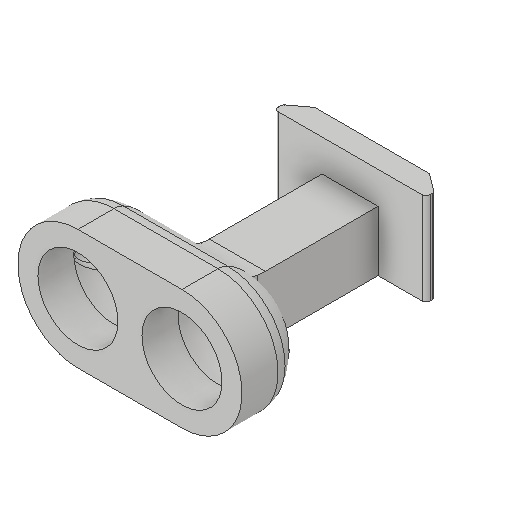
# Autodesk Inventor part: Engate CNMF NEM355-5.50
Saved by Autodesk Inventor 2026.2 (Build 302298010, 298A)
## iProperties
Manager: MANUTENÇÃO GUIFÕES - CP
Company: CP
Created: 2025-09-02
Part Number: Engate CNMF NEM355-5.50
Project: 0.00 0000/00
Checked By: PMFIGUEIREDO
Engr Approved By: JSSILVA
Material: Generic
Description: NOME DA PEÇA
Document SubType Name: Modeling
Designer: TPMIRANDA
Engineer: ISO 2768 - m K
Authority: Nº DESENHO PELO QUAL FOI SUBSITUIDO
Stock Number: 00000-000
Density: 1 g/cm^3
Appearance: Default
Distância: 5,500 mm
Title: UME 3400
Subject: CAIXA, INTERIOR, SUPORTE,
Author: TPMIRANDA
Keywords: Caixa de comentários. Substituir texto, ou eliminar.
Comments: UQE2300 UQE2400 UTE2240 UDD9630 CARRUAGENS SIMAFE CARRUAGENS CAF CARRUAGENS ARCO
Revision Number: Nº DESENHO QUE SUBSTITUI
Autodesk Inventor part; units mm, degrees
ref_plane "XY Plane" through (0, 0, 0) normal (0, 0, 1) x (1, 0, 0)
sketch "Sketch1" plane through (0, 0, 0) normal (0, 0, 1) x (1, 0, 0)
  line L0 (-1.3, 0) -> (1.3, 0) construction
  line L1 (1.3, 0) -> (1.3, 2)
  line L2 (1.3, 0) -> (2.8, 0)
  line L3 (2.8, 0) -> (2.8, 0.9)
  line L4 (2.3, 0) -> (2.3, 0.9)
  arc A0 (2.8, 0.9) -> (2.7412, 1.1353) centre (2.3, 0.9) ccw
  arc A1 (2.7412, 1.1353) -> (1.3, 2) centre (1.3, 0.3667) ccw
  arc A2 (2.3, 0.9) -> (1.3, 1.5) centre (1.3, 0.3667) ccw
  line L5 (2.8, 0) -> (2.3, 0)
  line L6 (0, 0) -> (0, 3.0045)
  line L7 (2.05, 2) -> (2.3, 2)
  line L8 (2.3, 2) -> (2.3, 0)
  line L9 (2.3, 0) -> (2.05, 0)
  line L10 (2.05, 0) -> (2.05, 2)
  point P0 (2.05, 0)
  dimension "d0" = 2.6
  dimension "d4" = 0.9
  dimension "d6" = 2
  dimension "d7" = 0.5
  dimension "d40" = 2
  dimension "d97" = 0.5
  constraints: 22 end point, 6 point on circle, 4 point on line, 3 centre point, 3 horizontal, 2 coincident, 2 collinear, 2 parallel, 2 perpendicular, 2 tangent, 2 vertical, 1 concentric, 1 midpoint
  measures "d0" distance of L0.start L0.end
  measures "d4" distance of L4.start L4.end
  measures "d6" diameter of L4 L1
  measures "d7" radius of A0
  measures "d40" distance from line of L1.end L2
  measures "d97" diameter of L8 L10
revolve "Revolution1" add sketch "Sketch1" angle 360 about axis through (1.3, 0, 0) along (0, 1, 0) contours L1 A2 L10 L2 | L1 A1 L10 A2 | L10 A2 L4 L2 | L10 A1 L8 A2 | L4 L8 A1 A0 L3 L2
ref_plane "Work Plane1" through (0, 5.5, 0) normal (0, 1, 0) x (-1, 0, 0)
sketch "Sketch2" plane through (0, 5.5, 0) normal (0, 1, 0) x (-1, 0, 0)
  line L0 (0, -1.25) -> (-0.7, -1.25)
  line L1 (-0.7, -1.25) -> (-0.7, 0.25)
  line L2 (-0.7, 0.25) -> (0, 0.25)
  line L3 (0, 0.25) -> (0, -1.25)
  point P0 (0, 0)
  point P1 (0, -0.5)
  dimension "d10" = 1.5
  dimension "d11" = 1.4
  dimension "d74" = 0.5
  constraints: 8 end point, 2 parallel, 1 horizontal, 1 midpoint, 1 perpendicular, 1 point on line
  measures "d10" distance of L0.end L1.end
  measures "d11" diameter of L1 L3
  measures "d74" distance of point (0, -0.5) point (0, 0)
extrude "Extrusion1" add sketch "Sketch2" against normal up to surface (5.5 mm away)
ref_plane "Work Plane7" through (1.3, 0, 0) normal (1, 0, 0) x (0, 1, 0)
sketch "Sketch17" plane through (1.3, 0, 0) normal (1, 0, 0) x (0, 1, 0)
  line L0 (0, 1.5) -> (0.9, 1.5) projected
  arc A0 (1.1353, 1.4412) -> (0.9, 1.5) centre (0.9, 1) ccw projected
  arc A1 (1.1353, -1.4412) -> (1.1353, 1.4412) centre (0.3667, 0) ccw projected
  arc A2 (0.9, -1.5) -> (1.1353, -1.4412) centre (0.9, -1) ccw projected
  line L1 (0, -1.5) -> (0.9, -1.5) projected
  line L2 (0, -1.5) -> (0, 1.5) projected
  point P0 (0, 0)
  point P1 (0, -0.7483)
  point P2 (0, -1.3748)
extrude "Extrusion14" add sketch "Sketch17" against normal up to surface (1.3 mm away)
revolve "Revolution2" cut sketch "Sketch1" angle 360 about axis through (1.3, 0, 0) along (0, 1, 0) contours L1 A2 L10 L2 | L10 A2 L4 L2
revolve "Revolução3" cut sketch "Sketch1" angle 360 about axis through (2.05, 0, 0) along (0, 1, 0) contours L10 A2 L4 L2 | L10 A1 L8 A2 | L10 L7 L8 A1
sketch "Sketch15" plane through (0.9792, 0.5, -1.25) normal (0, 0, -1) x (-1, 0, 0)
  line L0 (0.9792, 5) -> (-0.9208, 5)
  line L1 (-0.9208, 5) -> (-0.9208, 5.2)
  line L2 (-0.9208, 5.2) -> (-0.1208, 5.8)
  line L3 (-0.1208, 5.8) -> (0.9792, 5.8)
  line L4 (0.9792, 5.8) -> (0.9792, 5)
  line L5 (0.2792, 5) -> (0.9792, 5) projected
  line L6 (0.9792, 5) -> (0.9792, 0.918) projected
  point P0 (0.9292, -0.4176)
  point P1 (0.9792, 0.918)
  point P2 (0.9792, 1)
  dimension "d77" = 3.8
  dimension "d78" = 0.8
  dimension "d79" = 2.2
  dimension "d80" = 0.2
  constraints: 10 end point, 2 perpendicular, 1 collinear, 1 horizontal, 1 parallel, 1 vertical, 1 other
  measures "d77" diameter of L1 L4
  measures "d78" distance between parallel lines of L3 L0
  measures "d79" diameter of L2.end L4
  measures "d80" distance of L0.end L1.end
extrude "Extrusion12" add sketch "Sketch15" against normal blind 2.3
sketch "Sketch8" plane through (1.3, 0, -0.525) normal (0, -1, 0) x (0.8950301, 0, -0.4460058)
  circle A0 centre (-1.0647, 0.056) radius 0.2
  line L0 (-1.1954, -0.5159) -> (-1.3977, -0.1099)
  line L1 (-2.3343, 1.7696) -> (-0.4611, -1.9895) construction
  line L2 (-2.1137, -0.4667) -> (1.6454, 1.4065) construction
  circle A1 centre (-0.2342, 0.4699) radius 1 construction
  circle A2 centre (-1.1865, -0.0047) radius 0.064
  point P0 (-1.3977, -0.1099)
  dimension "d37" = 0.4
  dimension "d95" = 0.128
  constraints: 2 centre point, 2 end point, 2 point on line, 2 tangent, 1 coincident, 1 collinear
  measures "d37" diameter of A0
  measures "d95" diameter of A2
sketch "Sketch9" plane through (0, 0, 0) normal (0, 0, 1) x (1, 0, 0)
  line L0 (0.372, 1.4649) -> (0.372, 0)
  arc A0 (0.5184, 1.8184) -> (0.372, 1.4649) centre (0.872, 1.4649) ccw
  line L1 (3.5184, 4.8184) -> (0.5184, 1.8184)
  line L2 (0.7, 5.5) -> (0.7, 1.418) construction
  line L3 (1.3, 2) -> (0.7, 2) construction
  point P0 (0.372, 0)
  point P1 (0, 0)
  point P2 (0, 0)
  point P3 (0.7, 2)
  point P4 (0.7, 0.9)
  dimension "d42" = 0.5
  dimension "d84" = 45
  dimension "d96" = 3
  constraints: 4 end point, 3 point on line, 2 coincident, 2 point on circle, 2 tangent, 1 centre point, 1 vertical
  measures "d42" radius of A0
  measures "d96" horizontal distance of L1.start L1.end
sweep "Sweep1" [suppressed]
fillet "Fillet2" radius 0.5 1 edges at (0.7, 1.8959, -0.5737)
fillet "Fillet2" radius 1 1 edges at (0.35, 1.9808, 0.25)
fillet "Arredondamento4" radius 0.1 4 edges at (2.0493, 1.1794, 0.25) (2.0493, 1.1794, -0.25) (2.0466, 1.7977, -0.25) (2.0466, 1.7977, 0.25)
mirror "Mirror1" about plane through (0, 0, 0) normal (1, 0, 0)
sketch "Sketch16" plane through (1.1, 6.3, 1.05) normal (0, 1, 0) x (1, 0, 0)
  line L0 (0, 2.3) -> (0, 0) construction
  line L1 (-2.2, 2.3) -> (-2.2, 0) construction
  line L2 (0, 1.15) -> (-2.2, 1.15) construction
  circle A0 centre (-1.1, 1.15) radius 0.65
  point P0 (-1.1, 1.05)
  dimension "d88" = 1.3
  constraints: 3 midpoint, 2 end point, 1 centre point
  measures "d88" diameter of A0
extrude "Extrusion13" [suppressed]
chamfer "Chanfro1" distance 0.25 angle 45 2 edges at (0, 6.3, 1.05) (0, 6.3, -1.25)
fillet "Fillet3" radius 0.1 6 edges at (1.9, 5.7, -0.1) (-1.9, 5.7, -0.1) (1.1, 6.3, -0.1) (-1.1, 6.3, -0.1) (1.9, 5.5, -0.1) (-1.9, 5.5, -0.1)
sketch "Sketch11" plane through (0.75, 3.7797, -1.25) normal (0, 0, 1) x (1, 0, 0)
  circle A0 centre (-0.75, -1.7797) radius 0.2
  point P0 (-0.75, -3.7797)
  dimension "d58" = 2
  dimension "d59" = 0.4
  constraints: 1 centre point, 1 vertical alignment
  measures "d58" distance of point (-0.75, -3.78) A0.centre
  measures "d59" diameter of A0
extrude "Extrusion8" add sketch "Sketch11" against normal blind 0.1 draft -45
sketch "Sketch12" plane through (1.25, 2.6275, -1.25) normal (0, 0, -1) x (-1, 0, 0)
  circle A0 centre (1.25, -0.6275) radius 0.1 construction
  line L0 (1.05, -0.6275) -> (0.7036, -0.8275)
  line L1 (0.7036, -0.8275) -> (0.7036, -0.4275)
  line L2 (0.7036, -0.4275) -> (1.05, -0.6275)
  circle A1 centre (1.25, -0.6275) radius 0.2 construction
  circle A2 centre (1.25, -0.6275) radius 0.4309 construction
  line L3 (0.8191, -0.6275) -> (1.25, -0.6275) construction
  point P0 (1.25, -2.6275)
  dimension "d62" = 0.4
  constraints: 8 end point, 2 horizontal alignment, 1 coincident, 1 horizontal, 1 point on line, 10 other
  measures "d62" distance of L0.end L1.end
extrude "Extrusion9" add sketch "Sketch12" along normal blind 0.1 draft -45
pattern_circular "Circular Pattern1" count 2 over 360 about axis through (0, 2, -1.25) along (0, 0, -1) of "Extrusion9"
pattern_of_one "Rectangular Pattern1"
sketch "Sketch13" plane through (0, 2, -1.35) normal (0, 0, -1) x (-1, 0, 0)
  circle A0 centre (0, 0) radius 0.2 projected
  point P0 (0, -2)
extrude "Extrusion10" cut sketch "Sketch13" against normal up to surface (0.1 mm away)
body "Solid1"
